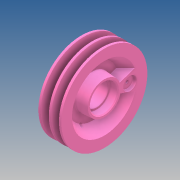
# Autodesk Inventor part: Carrete Impreso
Saved by Autodesk Inventor 2017 (Build 210142000, 142)
## iProperties
Part Number: Carrete Impreso
Material: Genérico
Document SubType Name: Modeling
Designer: Leo
Density: 1 g/cm^3
Appearance: Rosado
Author: Leo
Autodesk Inventor part; units mm, degrees
ref_plane "YZ Plane" through (0, 0, 0) normal (1, 0, 0) x (0, 1, 0)
sketch "Boceto1" plane through (0, 0, 0) normal (0, 0, 1) x (1, 0, 0)
  line L0 (-52.726, 0) -> (52.726, 0)
  line L1 (-7, 12.25) -> (7, 12.25)
  line L2 (7, 12.25) -> (7, 14.25)
  line L3 (7, 14.25) -> (15, 14.25)
  line L4 (15, 45) -> (12.5, 45)
  line L5 (12.5, 45) -> (10.9438, 36.8577)
  line L6 (-4.7765, 36.8915) -> (-6.5, 45)
  line L7 (-6.5, 45) -> (-9, 45)
  line L8 (-9, 45) -> (-9, 18.25)
  line L9 (-9, 18.25) -> (-15, 18.25)
  line L10 (-15, 18.25) -> (-15, 14.25)
  line L11 (-15, 14.25) -> (-7, 14.25)
  line L12 (-7, 14.25) -> (-7, 12.25)
  line L13 (15, 17.25) -> (2.7902, 18.25)
  line L14 (2.7902, 18.25) -> (2.7902, 26.25)
  line L15 (2.7902, 26.25) -> (15, 33.7899)
  line L16 (15, 14.25) -> (15, 17.25)
  line L17 (15, 33.7899) -> (15, 45)
  line L18 (7.6167, 22.25) -> (-2.0363, 22.25) construction
  line L19 (-15, 6) -> (-7, 6)
  line L20 (-7, 6) -> (-7, 8)
  line L21 (-7, 8) -> (7, 8)
  line L22 (7, 8) -> (7, 6)
  line L23 (7, 6) -> (15, 6)
  line L24 (15, 6) -> (15, 4)
  line L25 (15, 4) -> (-15, 4)
  line L26 (-15, 4) -> (-15, 6)
  arc A0 (6.4794, 36.7292) -> (10.9438, 36.8577) centre (8.6974, 37.2871) ccw
  line L27 (6.4794, 36.7292) -> (4.3992, 45)
  line L28 (4.3992, 45) -> (1.8992, 45)
  line L29 (1.8992, 45) -> (-0.332, 36.7686)
  arc A1 (-4.7765, 36.8915) -> (-0.332, 36.7686) centre (-2.5394, 37.367) ccw
  point P0 (0, 0)
  point P1 (0, 0)
  point P2 (0, 12.25)
  point P3 (2.7902, 22.25)
  point P4 (0, 4)
  dimension "d0" = 8
  dimension "d1" = 28.5
  dimension "d2" = 24.5
  dimension "d3" = 6
  dimension "d4" = 4
  dimension "d5" = 90
  dimension "d7" = 2.5
  dimension "d18" = 8
  dimension "d20" = 12
  dimension "d24" = 44.5
  dimension "d26" = 8
  dimension "d27" = 12
  dimension "d28" = 16
  dimension "d29" = 8
  dimension "d31" = 24
  dimension "d32" = 30
  dimension "d33" = 17.7902
  dimension "d52" = 4
  dimension "d53" = 70
  dimension "d54" = 3
  constraints: 60 end point, 14 perpendicular, 7 equal length, 5 horizontal, 5 midpoint, 5 point on line, 4 point on circle, 4 tangent, 4 vertical, 2 centre point, 2 collinear, 2 vertical alignment, 1 coincident, 1 equal radius
  measures "d0" distance of L10.end L11.end
  measures "d1" diameter of L11 L0
  measures "d2" diameter of L1 L0
  measures "d3" distance of L8.end L9.end
  measures "d4" distance of L9.end L10.end
  measures "d5" diameter of L4 L0
  measures "d7" distance of L6.end L7.end
  measures "d18" distance of L13.end L14.end
  measures "d20" angle of L8 L6
  measures "d24" diameter of L18 L0
  measures "d26" diameter of L25 L0
  measures "d27" diameter of L19 L0
  measures "d28" diameter of L21 L0
  measures "d29" distance of L19.start L19.end
  measures "d31" distance of L4.start L7.end
  measures "d32" distance of L24.end L25.end
  measures "d33" distance between parallel lines of L14 L10
  measures "d52" distance edge to line of A0 L15
  measures "d54" distance of L3.end L13.start
revolve "Revolución1" add sketch "Boceto1" angle 360 about axis through (-52.726, 0, 0) along (1, 0, 0) contours L12 L11 L10 L9 L8 L7 L6 A1 L29 L28 L27 A0 L5 L4 L17 L15 L14 L13 L16 L3 L2 L1
sketch "Boceto2" plane through (-15, 0, 0) normal (-1, 0, 0) x (0, 0, 1)
  circle A0 centre (0, 0) radius 18.25 projected
  arc A1 (-17.783, 20.168) -> (-26.3575, 5.3165) centre (-19.7021, 11.375) ccw
  arc A2 (-17.783, 20.168) -> (17.783, 20.168) centre (0, 101.6471) ccw
  arc A3 (26.3575, 5.3165) -> (17.783, 20.168) centre (19.7021, 11.375) ccw
  arc A4 (26.3575, 5.3165) -> (8.5745, -25.4845) centre (88.0289, -50.8235) ccw
  arc A5 (-8.5745, -25.4845) -> (8.5745, -25.4845) centre (0, -22.75) ccw
  arc A6 (-8.5745, -25.4845) -> (-26.3575, 5.3165) centre (-88.0289, -50.8235) ccw
  line L0 (-23.1662, -13.375) -> (19.7021, 11.375) construction
  line L1 (23.1662, -13.375) -> (-19.7021, 11.375) construction
  circle A7 centre (-19.7021, 11.375) radius 1.5 construction
  circle A8 centre (19.7021, 11.375) radius 1.5 construction
  circle A9 centre (23.1662, -13.375) radius 1.5
  circle A10 centre (-23.1662, -13.375) radius 1.5
  line L2 (0, 26.75) -> (0, -22.75) construction
  circle A11 centre (0, 26.75) radius 1.5
  circle A12 centre (0, -22.75) radius 1.5 construction
  point P0 (0, 0)
  point P1 (0, 0)
  dimension "d10" = 9
  dimension "d11" = 3
  dimension "d13" = 52.5
  dimension "d25" = 49.5
  dimension "d56" = 120
  dimension "d65" = 7
  dimension "d66" = 3
  dimension "d67" = 7
  dimension "d68" = 7
  constraints: 12 centre point, 12 point on circle, 9 tangent, 8 coincident, 7 equal radius, 6 end point, 3 point on line, 2 equal length, 1 horizontal alignment, 1 vertical
  measures "d10" radius of A1
  measures "d11" diameter of A7
  measures "d25" distance of L2.start L2.end
  measures "d56" angle of L0 L1
extrude "Extrusión1" add sketch "Boceto2" against normal up to next contours A0 A2 A3 A4 | A0 A6 A1 A2 | A4 A5 A6 A0
chamfer "Chaflán1" distance 1 angle 45 2 edges at (-15, -14.25, 0) (15, -14.25, 0)
sketch "Boceto4" plane through (0, 0, 0) normal (0, 0, 1) x (1, 0, 0)
  line L0 (15, 33.7899) -> (2.7902, 26.25)
  line L1 (2.7902, 18.25) -> (15, 17.25) construction
  line L2 (15, 33.7899) -> (15, 15.9306)
  line L3 (2.7902, 26.25) -> (2.7902, 15.9306)
  line L4 (-21, 0) -> (21, 0)
  line L5 (15, 15.9306) -> (2.7902, 15.9306)
  line L6 (-29.4, 0) -> (29.4, 0) projected
  point P0 (0, 0)
  constraints: 12 end point, 2 point on line, 1 horizontal
revolve "Revolución6" add sketch "Boceto4" angle 40 mid plane about axis through (-10, 0, 0) along (1, 0, 0)
extrude "Extrusión2" cut sketch "Boceto2" against normal through all contours A9 | A10 | A11
ref_plane "Plano de trabajo1" through (0, 0, 0) normal (0, -0.8660254, 0.5) x (1, 0, 0)
sketch "Boceto3" plane through (15, 0, 0) normal (1, 0, 0) x (0, 0, -1)
  line L0 (4.7815, 26.75) -> (2.3908, 22.6091)
  line L1 (2.3908, 22.6091) -> (-2.3908, 22.6091)
  line L2 (-2.3908, 22.6091) -> (-4.7815, 26.75)
  line L3 (-4.7815, 26.75) -> (-2.3908, 30.8909)
  line L4 (-2.3908, 30.8909) -> (2.3908, 30.8909)
  line L5 (2.3908, 30.8909) -> (4.7815, 26.75)
  circle A0 centre (0, 0) radius 26.25 construction
  circle A1 centre (0, 0) radius 18.25 construction
  circle A2 centre (0, 26.75) radius 1.5 projected
  circle A3 centre (0, 26.75) radius 6
  point P0 (0, 0)
  dimension "d34" = 8.2818
  dimension "d69" = 12
  dimension "d44" = 1.5
  constraints: 12 end point, 3 centre point, 2 coincident, 1 horizontal, 13 other
  measures "d34" distance between parallel lines of L4 L1
  measures "d69" diameter of A3
extrude "Extrusión3" cut sketch "Boceto3" against normal blind 3 contours L0 L1 L2 L3 L4 L5 | A2 | A3
chamfer "Chaflán2" distance 1 distance2 3 1 edges at (15, 26.75, 6) measured on face at (15, 26.75, 6.5)
chamfer "Chaflán3" distance 12.2 distance2 2 1 edges at (15, 23.9809, -8.7283) measured on face at (14.5, 23.9809, -8.7283)
chamfer "Chaflán4" [suppressed]
fillet "Empalme1" [suppressed]
